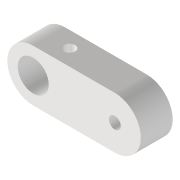
# Autodesk Inventor part: Holisheet_NEMA8_Syringe_pusher
Saved by Autodesk Inventor 2022 (Build 260153000, 153)
## iProperties
Created: 2023-03-11
Part Number: Holisheet_NEMA8_Syringe_pusher
Material: Generisch
Document SubType Name: Modeling
Designer: diederichbenedict
Density: 1 g/cm^3
Appearance: Vorgabe
Author: diederichbenedict
Autodesk Inventor part; units mm, degrees
ref_plane "YZ Plane" through (0, 0, 0) normal (1, 0, 0) x (0, 1, 0)
ref_plane "XZ Plane" through (0, 0, 0) normal (0, 1, 0) x (-1, 0, 0)
ref_plane "XY Plane" through (0, 0, 0) normal (0, 0, 1) x (1, 0, 0)
sketch "Skizze1" plane through (0, 0, 0) normal (0, 0, 1) x (1, 0, 0)
  circle A0 centre (0, 0) radius 1.5
  circle A1 centre (-20.5, 0) radius 1.8 projected
  circle A2 centre (-20.5, 0) radius 3.9
  line L0 (0, 0) -> (-20.5, 0) construction
  line L1 (0, 6.5) -> (-20.5, 6.5)
  line L2 (-20.5, -6.5) -> (0, -6.5)
  arc A3 (0, -6.5) -> (0, 6.5) centre (0, 0) ccw
  arc A4 (-20.5, 6.5) -> (-20.5, -6.5) centre (-20.5, 0) ccw
  point P0 (-10.25, 0)
  dimension "d0" = 3
  dimension "d1" = 7.8
  dimension "d2" = 13
  constraints: 8 end point, 4 centre point, 4 point on circle, 4 tangent, 2 coincident, 1 horizontal, 1 midpoint, 1 parallel
  measures "d0" diameter of A0
  measures "d1" diameter of A2
  measures "d2" diameter of A4
extrude "Extrusion1" add sketch "Skizze1" along normal blind 8 contours A3 L2 A4 L1
sketch "Skizze2" plane through (0, 0, 0) normal (0, 0, -1) x (-1, 0, 0)
  circle A0 centre (0, 0) radius 1.5 projected
  circle A1 centre (0, 0) radius 3.5
  dimension "d5" = 7
  constraints: 1 centre point, 1 coincident
  measures "d5" diameter of A1
extrude "Extrusion2" cut sketch "Skizze2" against normal blind 6 contours A0 | A1
sketch "Skizze3" plane through (-20.5, 6.5, 0) normal (0, 1, 0) x (1, 0, 0)
  line L0 (3.9, -8) -> (3.9, 0) projected
  circle A0 centre (5.1112, -4) radius 1.4
  point P0 (20.5, 0)
  dimension "d8" = 2.8
  constraints: 1 centre point
  measures "d8" diameter of A0
extrude "Extrusion3" cut sketch "Skizze3" against normal through all
